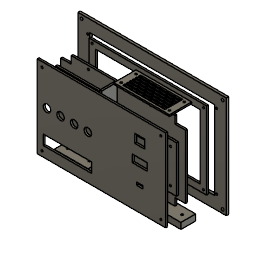
SmartMeter_Vista_Interna (Autodesk Fusion 360 design; units mm, degrees)
Autodesk Fusion 360 part; units mm, degrees
(part 1 of 2)
sketch "Esboço1" plane through (0, 0, 0) normal (0, 0, 1) x (1, 0, 0) in component "SmartMeter_DesktopFeet"
  line L0 (-102.5, -12) -> (-47.5, -12)
  line L1 (-47.5, -12) -> (-47.5, 12)
  line L2 (-47.5, 12) -> (-102.5, 12)
  line L3 (-102.5, 12) -> (-102.5, -12)
extrude "01_new_rect (1)" add sketch "Esboço1" along normal blind 10 makes body 1 in component "SmartMeter_DesktopFeet"
sketch "Esboço2" plane through (0, 0, 0) normal (0, 0, 1) x (1, 0, 0) in component "SmartMeter_DesktopFeet"
  circle A0 centre (-92.5, 0) radius 1.6
extrude "02_cut_circle (1)" cut sketch "Esboço2" along normal blind 11 bodies 1 in component "SmartMeter_DesktopFeet"
sketch "Esboço3" plane through (0, 0, 0) normal (0, 0, 1) x (1, 0, 0) in component "SmartMeter_DesktopFeet"
  circle A0 centre (-57.5, 0) radius 1.6
extrude "03_cut_circle (1)" cut sketch "Esboço3" along normal blind 11 bodies 1 in component "SmartMeter_DesktopFeet"
sketch "Esboço4" plane through (0, 0, 0) normal (0, 0, 1) x (1, 0, 0) in component "SmartMeter_DesktopFeet"
  line L0 (47.5, -12) -> (102.5, -12)
  line L1 (102.5, -12) -> (102.5, 12)
  line L2 (102.5, 12) -> (47.5, 12)
  line L3 (47.5, 12) -> (47.5, -12)
extrude "04_new_rect (1)" add sketch "Esboço4" along normal blind 10 separate body makes body 2 in component "SmartMeter_DesktopFeet"
sketch "Esboço5" plane through (0, 0, 0) normal (0, 0, 1) x (1, 0, 0) in component "SmartMeter_DesktopFeet"
  circle A0 centre (57.5, 0) radius 1.6
extrude "05_cut_circle (1)" cut sketch "Esboço5" along normal blind 11 bodies 1 2 in component "SmartMeter_DesktopFeet"
sketch "Esboço6" plane through (0, 0, 0) normal (0, 0, 1) x (1, 0, 0) in component "SmartMeter_DesktopFeet"
  circle A0 centre (92.5, 0) radius 1.6
extrude "06_cut_circle (1)" cut sketch "Esboço6" along normal blind 11 bodies 1 2 in component "SmartMeter_DesktopFeet"
sketch "Esboço1 (2)" plane through (0, 0, 0) normal (0, 0, 1) x (1, 0, 0) in component "SmartMeter_DisplayBracket"
  line L0 (-95, -62.5) -> (95, -62.5)
  line L1 (95, -62.5) -> (95, 62.5)
  line L2 (95, 62.5) -> (-95, 62.5)
  line L3 (-95, 62.5) -> (-95, -62.5)
extrude "01_new_rect (1)'" add sketch "Esboço1 (2)" along normal blind 3 separate body makes body 3 in component "SmartMeter_DisplayBracket"
sketch "Esboço2 (2)" plane through (0, 0, 0) normal (0, 0, 1) x (1, 0, 0) in component "SmartMeter_DisplayBracket"
  line L0 (-84.5, -52) -> (84.5, -52)
  line L1 (84.5, -52) -> (84.5, 52)
  line L2 (84.5, 52) -> (-84.5, 52)
  line L3 (-84.5, 52) -> (-84.5, -52)
extrude "02_cut_rect (1)" cut sketch "Esboço2 (2)" along normal blind 4 bodies 3 in component "SmartMeter_DisplayBracket"
sketch "Esboço3 (2)" plane through (0, 0, 0) normal (0, 0, 1) x (1, 0, 0) in component "SmartMeter_DisplayBracket"
  line L0 (-12, -62.5) -> (12, -62.5)
  line L1 (12, -62.5) -> (12, -52.5)
  line L2 (12, -52.5) -> (-12, -52.5)
  line L3 (-12, -52.5) -> (-12, -62.5)
extrude "03_cut_rect (1)" cut sketch "Esboço3 (2)" along normal blind 4 bodies 3 in component "SmartMeter_DisplayBracket"
sketch "Esboço4 (2)" plane through (0, 0, 0) normal (0, 0, 1) x (1, 0, 0) in component "SmartMeter_DisplayBracket"
  circle A0 centre (-90, -57.5) radius 1.6
extrude "04_cut_circle (1)" cut sketch "Esboço4 (2)" along normal blind 4 bodies 3 in component "SmartMeter_DisplayBracket"
sketch "Esboço5 (2)" plane through (0, 0, 0) normal (0, 0, 1) x (1, 0, 0) in component "SmartMeter_DisplayBracket"
  circle A0 centre (-90, 57.5) radius 1.6
extrude "05_cut_circle (1)'" cut sketch "Esboço5 (2)" along normal blind 4 bodies 3 in component "SmartMeter_DisplayBracket"
sketch "Esboço6 (2)" plane through (0, 0, 0) normal (0, 0, 1) x (1, 0, 0) in component "SmartMeter_DisplayBracket"
  circle A0 centre (90, -57.5) radius 1.6
extrude "06_cut_circle (1)'" cut sketch "Esboço6 (2)" along normal blind 4 bodies 3 in component "SmartMeter_DisplayBracket"
sketch "Esboço7" plane through (0, 0, 0) normal (0, 0, 1) x (1, 0, 0) in component "SmartMeter_DisplayBracket"
  circle A0 centre (90, 57.5) radius 1.6
extrude "07_cut_circle (1)" cut sketch "Esboço7" along normal blind 4 bodies 3 in component "SmartMeter_DisplayBracket"
sketch "Esboço1 (3)" plane through (0, 0, 0) normal (0, 0, 1) x (1, 0, 0) in component "SmartMeter_FrontPanel"
  line L0 (-102, 72.5) -> (102, 72.5)
  arc A0 (110, 64.5) -> (102, 72.5) centre (102, 64.5) ccw
  line L1 (110, 64.5) -> (110, -64.5)
  arc A1 (102, -72.5) -> (110, -64.5) centre (102, -64.5) ccw
  line L2 (102, -72.5) -> (-102, -72.5)
  arc A2 (-110, -64.5) -> (-102, -72.5) centre (-102, -64.5) ccw
  line L3 (-110, -64.5) -> (-110, 64.5)
  arc A3 (-102, 72.5) -> (-110, 64.5) centre (-102, 64.5) ccw
extrude "01_new_rounded (1)" add sketch "Esboço1 (3)" along normal blind 4 separate body makes body 4 in component "SmartMeter_FrontPanel"
sketch "Esboço2 (3)" plane through (0, 0, 0) normal (0, 0, 1) x (1, 0, 0) in component "SmartMeter_FrontPanel"
  line L0 (-77.5, -43.5) -> (77.5, -43.5)
  line L1 (77.5, -43.5) -> (77.5, 43.5)
  line L2 (77.5, 43.5) -> (-77.5, 43.5)
  line L3 (-77.5, 43.5) -> (-77.5, -43.5)
extrude "02_cut_rect (1)'" cut sketch "Esboço2 (3)" along normal blind 5 bodies 4 in component "SmartMeter_FrontPanel"
ref_plane "Plano de trabalho1" through (0, 0, 1.5) normal (0, 0, 1) x (1, 0, 0) in component "SmartMeter_FrontPanel"
sketch "Esboço3 (3)" plane through (0, 0, 1.5) normal (0, 0, 1) x (1, 0, 0) in component "SmartMeter_FrontPanel"
  line L0 (-83.5, -51) -> (83.5, -51)
  line L1 (83.5, -51) -> (83.5, 51)
  line L2 (83.5, 51) -> (-83.5, 51)
  line L3 (-83.5, 51) -> (-83.5, -51)
extrude "03_cut_rect (1)'" cut sketch "Esboço3 (3)" along normal blind 2.7 bodies 4 in component "SmartMeter_FrontPanel"
sketch "Esboço4 (3)" plane through (0, 0, 0) normal (0, 0, 1) x (1, 0, 0) in component "SmartMeter_FrontPanel"
  circle A0 centre (-90, -57.5) radius 1.6
extrude "04_cut_circle (1)'" cut sketch "Esboço4 (3)" along normal blind 5 bodies 4 in component "SmartMeter_FrontPanel"
sketch "Esboço5 (3)" plane through (0, 0, 0) normal (0, 0, 1) x (1, 0, 0) in component "SmartMeter_FrontPanel"
  circle A0 centre (-90, 57.5) radius 1.6
extrude "05_cut_circle (1)''" cut sketch "Esboço5 (3)" along normal blind 5 bodies 4 in component "SmartMeter_FrontPanel"
sketch "Esboço6 (3)" plane through (0, 0, 0) normal (0, 0, 1) x (1, 0, 0) in component "SmartMeter_FrontPanel"
  circle A0 centre (90, -57.5) radius 1.6
extrude "06_cut_circle (1)''" cut sketch "Esboço6 (3)" along normal blind 5 bodies 4 in component "SmartMeter_FrontPanel"
sketch "Esboço7 (2)" plane through (0, 0, 0) normal (0, 0, 1) x (1, 0, 0) in component "SmartMeter_FrontPanel"
  circle A0 centre (90, 57.5) radius 1.6
extrude "07_cut_circle (1)'" cut sketch "Esboço7 (2)" along normal blind 5 bodies 4 in component "SmartMeter_FrontPanel"
sketch "Esboço8" plane through (0, 0, 0) normal (0, 0, 1) x (1, 0, 0) in component "SmartMeter_FrontPanel"
  circle A0 centre (-104, -60) radius 1.6
extrude "08_cut_circle (1)" cut sketch "Esboço8" along normal blind 4 bodies 4 in component "SmartMeter_FrontPanel"
sketch "Esboço9" plane through (0, 0, 0) normal (0, 0, 1) x (1, 0, 0) in component "SmartMeter_FrontPanel"
  circle A0 centre (-104, 60) radius 1.6
extrude "09_cut_circle (1)" cut sketch "Esboço9" along normal blind 4 bodies 4 in component "SmartMeter_FrontPanel"
sketch "Esboço10" plane through (0, 0, 0) normal (0, 0, 1) x (1, 0, 0) in component "SmartMeter_FrontPanel"
  circle A0 centre (104, -60) radius 1.6
extrude "10_cut_circle (1)" cut sketch "Esboço10" along normal blind 4 bodies 4 in component "SmartMeter_FrontPanel"
sketch "Esboço11" plane through (0, 0, 0) normal (0, 0, 1) x (1, 0, 0) in component "SmartMeter_FrontPanel"
  circle A0 centre (104, 60) radius 1.6
extrude "11_cut_circle (1)" cut sketch "Esboço11" along normal blind 4 bodies 4 in component "SmartMeter_FrontPanel"
sketch "Esboço1 (4)" plane through (0, 0, 0) normal (0, 0, 1) x (1, 0, 0) in component "SmartMeter_InternalTray"
  line L0 (-101, -63.5) -> (101, -63.5)
  line L1 (101, -63.5) -> (101, 63.5)
  line L2 (101, 63.5) -> (-101, 63.5)
  line L3 (-101, 63.5) -> (-101, -63.5)
extrude "01_new_rect (1)''" add sketch "Esboço1 (4)" along normal blind 3 separate body makes body 5 in component "SmartMeter_InternalTray"
sketch "Esboço2 (4)" plane through (0, 0, 0) normal (0, 0, 1) x (1, 0, 0) in component "SmartMeter_InternalTray"
  line L0 (-12.5, -63.5) -> (-9.5, -63.5)
  line L1 (-9.5, -63.5) -> (-9.5, 63.5)
  line L2 (-9.5, 63.5) -> (-12.5, 63.5)
  line L3 (-12.5, 63.5) -> (-12.5, -63.5)
extrude "Extrusão2" add sketch "Esboço2 (4)" along normal blind 28 separate body makes body 6 in component "SmartMeter_InternalTray"
combine "02_join_rect (1)" operation add target body 5 tool bodies 6 in component "SmartMeter_InternalTray"
sketch "Esboço3 (4)" plane through (0, 0, 0) normal (0, 0, 1) x (1, 0, 0) in component "SmartMeter_InternalTray"
  circle A0 centre (-86, -30) radius 5
extrude "Extrusão3" add sketch "Esboço3 (4)" along normal blind 11 separate body makes body 7 in component "SmartMeter_InternalTray"
combine "03_join_circle (1)" operation add target body 5 tool bodies 7 in component "SmartMeter_InternalTray"
sketch "Esboço4 (4)" plane through (0, 0, 0) normal (0, 0, 1) x (1, 0, 0) in component "SmartMeter_InternalTray"
  circle A0 centre (-86, 30) radius 5
extrude "Extrusão4" add sketch "Esboço4 (4)" along normal blind 11 separate body makes body 8 in component "SmartMeter_InternalTray"
combine "04_join_circle (1)" operation add target body 5 tool bodies 8 in component "SmartMeter_InternalTray"
sketch "Esboço5 (4)" plane through (0, 0, 0) normal (0, 0, 1) x (1, 0, 0) in component "SmartMeter_InternalTray"
  circle A0 centre (-26, -30) radius 5
extrude "Extrusão5" add sketch "Esboço5 (4)" along normal blind 11 separate body makes body 9 in component "SmartMeter_InternalTray"
combine "05_join_circle (1)" operation add target body 5 tool bodies 9 in component "SmartMeter_InternalTray"
sketch "Esboço6 (4)" plane through (0, 0, 0) normal (0, 0, 1) x (1, 0, 0) in component "SmartMeter_InternalTray"
  circle A0 centre (-26, 30) radius 5
extrude "Extrusão6" add sketch "Esboço6 (4)" along normal blind 11 separate body makes body 10 in component "SmartMeter_InternalTray"
combine "06_join_circle (1)" operation add target body 5 tool bodies 10 in component "SmartMeter_InternalTray"
sketch "Esboço7 (3)" plane through (0, 0, 0) normal (0, 0, 1) x (1, 0, 0) in component "SmartMeter_InternalTray"
  circle A0 centre (10, -25) radius 5
extrude "Extrusão7" add sketch "Esboço7 (3)" along normal blind 11 separate body makes body 11 in component "SmartMeter_InternalTray"
combine "07_join_circle (1)" operation add target body 5 tool bodies 11 in component "SmartMeter_InternalTray"
sketch "Esboço8 (2)" plane through (0, 0, 0) normal (0, 0, 1) x (1, 0, 0) in component "SmartMeter_InternalTray"
  circle A0 centre (10, 25) radius 5
extrude "Extrusão8" add sketch "Esboço8 (2)" along normal blind 11 separate body makes body 12 in component "SmartMeter_InternalTray"
combine "08_join_circle (1)" operation add target body 5 tool bodies 12 in component "SmartMeter_InternalTray"
sketch "Esboço9 (2)" plane through (0, 0, 0) normal (0, 0, 1) x (1, 0, 0) in component "SmartMeter_InternalTray"
  circle A0 centre (80, -25) radius 5
extrude "Extrusão9" add sketch "Esboço9 (2)" along normal blind 11 separate body makes body 13 in component "SmartMeter_InternalTray"
combine "09_join_circle (1)" operation add target body 5 tool bodies 13 in component "SmartMeter_InternalTray"
sketch "Esboço10 (2)" plane through (0, 0, 0) normal (0, 0, 1) x (1, 0, 0) in component "SmartMeter_InternalTray"
  circle A0 centre (80, 25) radius 5
extrude "Extrusão10" add sketch "Esboço10 (2)" along normal blind 11 separate body makes body 14 in component "SmartMeter_InternalTray"
combine "10_join_circle (1)" operation add target body 5 tool bodies 14 in component "SmartMeter_InternalTray"
sketch "Esboço11 (2)" plane through (0, 0, 0) normal (0, 0, 1) x (1, 0, 0) in component "SmartMeter_InternalTray"
  line L0 (-28.5, -12) -> (-20.5, -12)
  line L1 (-20.5, -12) -> (-20.5, 12)
  line L2 (-20.5, 12) -> (-28.5, 12)
  line L3 (-28.5, 12) -> (-28.5, -12)
extrude "11_cut_rect (1)" cut sketch "Esboço11 (2)" along normal blind 3 bodies 5 in component "SmartMeter_InternalTray"
sketch "Esboço12" plane through (0, 0, 0) normal (0, 0, 1) x (1, 0, 0) in component "SmartMeter_InternalTray"
  line L0 (-1.5, -12) -> (6.5, -12)
  line L1 (6.5, -12) -> (6.5, 12)
  line L2 (6.5, 12) -> (-1.5, 12)
  line L3 (-1.5, 12) -> (-1.5, -12)
extrude "12_cut_rect (1)" cut sketch "Esboço12" along normal blind 3 bodies 5 in component "SmartMeter_InternalTray"
ref_plane "Plano de trabalho1" through (0, 0, 3) normal (0, 0, 1) x (1, 0, 0) in component "SmartMeter_InternalTray"
sketch "Esboço13" plane through (0, 0, 3) normal (0, 0, 1) x (1, 0, 0) in component "SmartMeter_InternalTray"
  circle A0 centre (-86, -30) radius 1.6
extrude "13_cut_circle (1)" cut sketch "Esboço13" along normal blind 8 bodies 5 in component "SmartMeter_InternalTray"
ref_plane "Plano de trabalho2" through (0, 0, 3) normal (0, 0, 1) x (1, 0, 0) in component "SmartMeter_InternalTray"
sketch "Esboço14" plane through (0, 0, 3) normal (0, 0, 1) x (1, 0, 0) in component "SmartMeter_InternalTray"
  circle A0 centre (-86, 30) radius 1.6
extrude "14_cut_circle (1)" cut sketch "Esboço14" along normal blind 8 bodies 5 in component "SmartMeter_InternalTray"
ref_plane "Plano de trabalho3" through (0, 0, 3) normal (0, 0, 1) x (1, 0, 0) in component "SmartMeter_InternalTray"
sketch "Esboço15" plane through (0, 0, 3) normal (0, 0, 1) x (1, 0, 0) in component "SmartMeter_InternalTray"
  circle A0 centre (-26, -30) radius 1.6
extrude "15_cut_circle (1)" cut sketch "Esboço15" along normal blind 8 bodies 5 in component "SmartMeter_InternalTray"
ref_plane "Plano de trabalho4" through (0, 0, 3) normal (0, 0, 1) x (1, 0, 0) in component "SmartMeter_InternalTray"
sketch "Esboço16" plane through (0, 0, 3) normal (0, 0, 1) x (1, 0, 0) in component "SmartMeter_InternalTray"
  circle A0 centre (-26, 30) radius 1.6
extrude "16_cut_circle (1)" cut sketch "Esboço16" along normal blind 8 bodies 5 in component "SmartMeter_InternalTray"
ref_plane "Plano de trabalho5" through (0, 0, 3) normal (0, 0, 1) x (1, 0, 0) in component "SmartMeter_InternalTray"
sketch "Esboço17" plane through (0, 0, 3) normal (0, 0, 1) x (1, 0, 0) in component "SmartMeter_InternalTray"
  circle A0 centre (10, -25) radius 1.6
extrude "17_cut_circle (1)" cut sketch "Esboço17" along normal blind 8 bodies 5 in component "SmartMeter_InternalTray"
ref_plane "Plano de trabalho6" through (0, 0, 3) normal (0, 0, 1) x (1, 0, 0) in component "SmartMeter_InternalTray"
sketch "Esboço18" plane through (0, 0, 3) normal (0, 0, 1) x (1, 0, 0) in component "SmartMeter_InternalTray"
  circle A0 centre (10, 25) radius 1.6
extrude "18_cut_circle (1)" cut sketch "Esboço18" along normal blind 8 bodies 5 in component "SmartMeter_InternalTray"
ref_plane "Plano de trabalho7" through (0, 0, 3) normal (0, 0, 1) x (1, 0, 0) in component "SmartMeter_InternalTray"
sketch "Esboço19" plane through (0, 0, 3) normal (0, 0, 1) x (1, 0, 0) in component "SmartMeter_InternalTray"
  circle A0 centre (80, -25) radius 1.6
extrude "19_cut_circle (1)" cut sketch "Esboço19" along normal blind 8 bodies 5 in component "SmartMeter_InternalTray"
ref_plane "Plano de trabalho8" through (0, 0, 3) normal (0, 0, 1) x (1, 0, 0) in component "SmartMeter_InternalTray"
sketch "Esboço20" plane through (0, 0, 3) normal (0, 0, 1) x (1, 0, 0) in component "SmartMeter_InternalTray"
  circle A0 centre (80, 25) radius 1.6
extrude "20_cut_circle (1)" cut sketch "Esboço20" along normal blind 8 bodies 5 in component "SmartMeter_InternalTray"
sketch "Esboço21" plane through (0, 0, 0) normal (0, 0, 1) x (1, 0, 0) in component "SmartMeter_InternalTray"
  line L0 (-101, -63.5) -> (-84, -63.5)
  line L1 (-84, -63.5) -> (-84, -51.5)
  line L2 (-84, -51.5) -> (-101, -51.5)
  line L3 (-101, -51.5) -> (-101, -63.5)
extrude "21_cut_rect (1)" cut sketch "Esboço21" along normal blind 3 bodies 5 in component "SmartMeter_InternalTray"
sketch "Esboço22" plane through (0, 0, 0) normal (0, 0, 1) x (1, 0, 0) in component "SmartMeter_InternalTray"
  line L0 (-101, 51.5) -> (-84, 51.5)
  line L1 (-84, 51.5) -> (-84, 63.5)
  line L2 (-84, 63.5) -> (-101, 63.5)
  line L3 (-101, 63.5) -> (-101, 51.5)
extrude "22_cut_rect (1)" cut sketch "Esboço22" along normal blind 3 bodies 5 in component "SmartMeter_InternalTray"
sketch "Esboço23" plane through (0, 0, 0) normal (0, 0, 1) x (1, 0, 0) in component "SmartMeter_InternalTray"
  line L0 (84, -63.5) -> (101, -63.5)
  line L1 (101, -63.5) -> (101, -51.5)
  line L2 (101, -51.5) -> (84, -51.5)
  line L3 (84, -51.5) -> (84, -63.5)
extrude "23_cut_rect (1)" cut sketch "Esboço23" along normal blind 3 bodies 5 in component "SmartMeter_InternalTray"
sketch "Esboço24" plane through (0, 0, 0) normal (0, 0, 1) x (1, 0, 0) in component "SmartMeter_InternalTray"
  line L0 (84, 51.5) -> (101, 51.5)
  line L1 (101, 51.5) -> (101, 63.5)
  line L2 (101, 63.5) -> (84, 63.5)
  line L3 (84, 63.5) -> (84, 51.5)
extrude "24_cut_rect (1)" cut sketch "Esboço24" along normal blind 3 bodies 5 in component "SmartMeter_InternalTray"
sketch "Esboço25" plane through (0, 0, 0) normal (0, 0, 1) x (1, 0, 0) in component "SmartMeter_InternalTray"
  circle A0 centre (-56, -58) radius 1.6
extrude "25_cut_circle (1)" cut sketch "Esboço25" along normal blind 3 bodies 5 in component "SmartMeter_InternalTray"
sketch "Esboço26" plane through (0, 0, 0) normal (0, 0, 1) x (1, 0, 0) in component "SmartMeter_InternalTray"
  circle A0 centre (-56, 58) radius 1.6
extrude "26_cut_circle (1)" cut sketch "Esboço26" along normal blind 3 bodies 5 in component "SmartMeter_InternalTray"
sketch "Esboço27" plane through (0, 0, 0) normal (0, 0, 1) x (1, 0, 0) in component "SmartMeter_InternalTray"
  circle A0 centre (45, -58) radius 1.6
extrude "27_cut_circle (1)" cut sketch "Esboço27" along normal blind 3 bodies 5 in component "SmartMeter_InternalTray"
sketch "Esboço28" plane through (0, 0, 0) normal (0, 0, 1) x (1, 0, 0) in component "SmartMeter_InternalTray"
  circle A0 centre (45, 58) radius 1.6
extrude "28_cut_circle (1)" cut sketch "Esboço28" along normal blind 3 bodies 5 in component "SmartMeter_InternalTray"
sketch "Esboço1 (5)" plane through (0, 0, 0) normal (0, 0, 1) x (1, 0, 0) in component "SmartMeter_PanelMountFrame"
  line L0 (-120, -82.5) -> (120, -82.5)
  line L1 (120, -82.5) -> (120, 82.5)
  line L2 (120, 82.5) -> (-120, 82.5)
  line L3 (-120, 82.5) -> (-120, -82.5)
extrude "01_new_rect (1)'''" add sketch "Esboço1 (5)" along normal blind 4 separate body makes body 15 in component "SmartMeter_PanelMountFrame"
sketch "Esboço2 (5)" plane through (0, 0, 0) normal (0, 0, 1) x (1, 0, 0) in component "SmartMeter_PanelMountFrame"
  line L0 (-101, -63.5) -> (101, -63.5)
  line L1 (101, -63.5) -> (101, 63.5)
  line L2 (101, 63.5) -> (-101, 63.5)
  line L3 (-101, 63.5) -> (-101, -63.5)
extrude "02_cut_rect (1)''" cut sketch "Esboço2 (5)" along normal blind 5 bodies 15 in component "SmartMeter_PanelMountFrame"
sketch "Esboço3 (5)" plane through (0, 0, 0) normal (0, 0, 1) x (1, 0, 0) in component "SmartMeter_PanelMountFrame"
  circle A0 centre (-114, -76.5) radius 2.25
extrude "03_cut_circle (1)'" cut sketch "Esboço3 (5)" along normal blind 5 bodies 15 in component "SmartMeter_PanelMountFrame"
sketch "Esboço4 (5)" plane through (0, 0, 0) normal (0, 0, 1) x (1, 0, 0) in component "SmartMeter_PanelMountFrame"
  circle A0 centre (-114, 76.5) radius 2.25
extrude "04_cut_circle (1)''" cut sketch "Esboço4 (5)" along normal blind 5 bodies 15 in component "SmartMeter_PanelMountFrame"
sketch "Esboço5 (5)" plane through (0, 0, 0) normal (0, 0, 1) x (1, 0, 0) in component "SmartMeter_PanelMountFrame"
  circle A0 centre (114, -76.5) radius 2.25
extrude "05_cut_circle (1)'''" cut sketch "Esboço5 (5)" along normal blind 5 bodies 15 in component "SmartMeter_PanelMountFrame"
sketch "Esboço6 (5)" plane through (0, 0, 0) normal (0, 0, 1) x (1, 0, 0) in component "SmartMeter_PanelMountFrame"
  circle A0 centre (114, 76.5) radius 2.25
extrude "06_cut_circle (1)'''" cut sketch "Esboço6 (5)" along normal blind 5 bodies 15 in component "SmartMeter_PanelMountFrame"
sketch "Esboço7 (4)" plane through (0, 0, 0) normal (0, 0, 1) x (1, 0, 0) in component "SmartMeter_PanelMountFrame"
  circle A0 centre (-104, -60) radius 1.6
extrude "07_cut_circle (1)''" cut sketch "Esboço7 (4)" along normal blind 4 bodies 15 in component "SmartMeter_PanelMountFrame"
sketch "Esboço8 (3)" plane through (0, 0, 0) normal (0, 0, 1) x (1, 0, 0) in component "SmartMeter_PanelMountFrame"
  circle A0 centre (-104, 60) radius 1.6
extrude "08_cut_circle (1)'" cut sketch "Esboço8 (3)" along normal blind 4 bodies 15 in component "SmartMeter_PanelMountFrame"
sketch "Esboço9 (3)" plane through (0, 0, 0) normal (0, 0, 1) x (1, 0, 0) in component "SmartMeter_PanelMountFrame"
  circle A0 centre (104, -60) radius 1.6
extrude "09_cut_circle (1)'" cut sketch "Esboço9 (3)" along normal blind 4 bodies 15 in component "SmartMeter_PanelMountFrame"
sketch "Esboço10 (3)" plane through (0, 0, 0) normal (0, 0, 1) x (1, 0, 0) in component "SmartMeter_PanelMountFrame"
  circle A0 centre (104, 60) radius 1.6
extrude "10_cut_circle (1)'" cut sketch "Esboço10 (3)" along normal blind 4 bodies 15 in component "SmartMeter_PanelMountFrame"
sketch "Esboço1 (6)" plane through (0, 0, 0) normal (0, 0, 1) x (1, 0, 0) in component "SmartMeter_RearHousing"
  line L0 (-110, -72.5) -> (110, -72.5)
  line L1 (110, -72.5) -> (110, 72.5)
  line L2 (110, 72.5) -> (-110, 72.5)
  line L3 (-110, 72.5) -> (-110, -72.5)
extrude "01_new_rect (1)''''" add sketch "Esboço1 (6)" along normal blind 75 separate body makes body 16 in component "SmartMeter_RearHousing"
sketch "Esboço2 (6)" plane through (0, 0, 0) normal (0, 0, 1) x (1, 0, 0) in component "SmartMeter_RearHousing"
  line L0 (-107, -69.5) -> (107, -69.5)
  line L1 (107, -69.5) -> (107, 69.5)
  line L2 (107, 69.5) -> (-107, 69.5)
  line L3 (-107, 69.5) -> (-107, -69.5)
extrude "02_cut_rect (1)'''" cut sketch "Esboço2 (6)" along normal blind 72 bodies 16 in component "SmartMeter_RearHousing"
ref_plane "Plano de trabalho1" through (0, 0, 3) normal (0, 0, 1) x (1, 0, 0) in component "SmartMeter_RearHousing"
sketch "Esboço3 (6)" plane through (0, 0, 3) normal (0, 0, 1) x (1, 0, 0) in component "SmartMeter_RearHousing"
  circle A0 centre (-90, -57.5) radius 5
extrude "Extrusão3'" add sketch "Esboço3 (6)" along normal blind 72 separate body makes body 17 in component "SmartMeter_RearHousing"
combine "03_join_circle (1)'" operation add target body 16 tool bodies 17 in component "SmartMeter_RearHousing"
ref_plane "Plano de trabalho2" through (0, 0, 3) normal (0, 0, 1) x (1, 0, 0) in component "SmartMeter_RearHousing"
sketch "Esboço4 (6)" plane through (0, 0, 3) normal (0, 0, 1) x (1, 0, 0) in component "SmartMeter_RearHousing"
  circle A0 centre (-90, 57.5) radius 5
extrude "Extrusão4'" add sketch "Esboço4 (6)" along normal blind 72 separate body makes body 18 in component "SmartMeter_RearHousing"
combine "04_join_circle (1)'" operation add target body 16 tool bodies 18 in component "SmartMeter_RearHousing"
ref_plane "Plano de trabalho3" through (0, 0, 3) normal (0, 0, 1) x (1, 0, 0) in component "SmartMeter_RearHousing"
sketch "Esboço5 (6)" plane through (0, 0, 3) normal (0, 0, 1) x (1, 0, 0) in component "SmartMeter_RearHousing"
  circle A0 centre (90, -57.5) radius 5
extrude "Extrusão5'" add sketch "Esboço5 (6)" along normal blind 72 separate body makes body 19 in component "SmartMeter_RearHousing"
combine "05_join_circle (1)'" operation add target body 16 tool bodies 19 in component "SmartMeter_RearHousing"
ref_plane "Plano de trabalho4" through (0, 0, 3) normal (0, 0, 1) x (1, 0, 0) in component "SmartMeter_RearHousing"
sketch "Esboço6 (6)" plane through (0, 0, 3) normal (0, 0, 1) x (1, 0, 0) in component "SmartMeter_RearHousing"
  circle A0 centre (90, 57.5) radius 5
extrude "Extrusão6'" add sketch "Esboço6 (6)" along normal blind 72 separate body makes body 20 in component "SmartMeter_RearHousing"
combine "06_join_circle (1)'" operation add target body 16 tool bodies 20 in component "SmartMeter_RearHousing"
ref_plane "Plano de trabalho5" through (0, 0, 3) normal (0, 0, 1) x (1, 0, 0) in component "SmartMeter_RearHousing"
sketch "Esboço7 (5)" plane through (0, 0, 3) normal (0, 0, 1) x (1, 0, 0) in component "SmartMeter_RearHousing"
  circle A0 centre (-90, -57.5) radius 2.3
extrude "07_cut_circle (1)'''" cut sketch "Esboço7 (5)" along normal blind 9 bodies 16 in component "SmartMeter_RearHousing"
ref_plane "Plano de trabalho6" through (0, 0, 3) normal (0, 0, 1) x (1, 0, 0) in component "SmartMeter_RearHousing"
sketch "Esboço8 (4)" plane through (0, 0, 3) normal (0, 0, 1) x (1, 0, 0) in component "SmartMeter_RearHousing"
  circle A0 centre (-90, 57.5) radius 2.3
extrude "08_cut_circle (1)''" cut sketch "Esboço8 (4)" along normal blind 9 bodies 16 in component "SmartMeter_RearHousing"
ref_plane "Plano de trabalho7" through (0, 0, 3) normal (0, 0, 1) x (1, 0, 0) in component "SmartMeter_RearHousing"
sketch "Esboço9 (4)" plane through (0, 0, 3) normal (0, 0, 1) x (1, 0, 0) in component "SmartMeter_RearHousing"
  circle A0 centre (90, -57.5) radius 2.3
extrude "09_cut_circle (1)''" cut sketch "Esboço9 (4)" along normal blind 9 bodies 16 in component "SmartMeter_RearHousing"
ref_plane "Plano de trabalho8" through (0, 0, 3) normal (0, 0, 1) x (1, 0, 0) in component "SmartMeter_RearHousing"
sketch "Esboço10 (4)" plane through (0, 0, 3) normal (0, 0, 1) x (1, 0, 0) in component "SmartMeter_RearHousing"
  circle A0 centre (90, 57.5) radius 2.3
extrude "10_cut_circle (1)''" cut sketch "Esboço10 (4)" along normal blind 9 bodies 16 in component "SmartMeter_RearHousing"
ref_plane "Plano de trabalho9" through (0, 0, 72) normal (0, 0, 1) x (1, 0, 0) in component "SmartMeter_RearHousing"
sketch "Esboço11 (3)" plane through (0, 0, 72) normal (0, 0, 1) x (1, 0, 0) in component "SmartMeter_RearHousing"
  line L0 (-94, -50) -> (-16, -50)
  line L1 (-16, -50) -> (-16, -34)
  line L2 (-16, -34) -> (-94, -34)
  line L3 (-94, -34) -> (-94, -50)
extrude "11_cut_rect (1)'" cut sketch "Esboço11 (3)" along normal blind 4 bodies 16 in component "SmartMeter_RearHousing"
ref_plane "Plano de trabalho10" through (0, 0, 72) normal (0, 0, 1) x (1, 0, 0) in component "SmartMeter_RearHousing"
sketch "Esboço12 (2)" plane through (0, 0, 72) normal (0, 0, 1) x (1, 0, 0) in component "SmartMeter_RearHousing"
  circle A0 centre (-88, 5) radius 6
extrude "12_cut_circle (1)" cut sketch "Esboço12 (2)" along normal blind 4 bodies 16 in component "SmartMeter_RearHousing"
ref_plane "Plano de trabalho11" through (0, 0, 72) normal (0, 0, 1) x (1, 0, 0) in component "SmartMeter_RearHousing"
sketch "Esboço13 (2)" plane through (0, 0, 72) normal (0, 0, 1) x (1, 0, 0) in component "SmartMeter_RearHousing"
  circle A0 centre (-66, 5) radius 6
extrude "13_cut_circle (1)'" cut sketch "Esboço13 (2)" along normal blind 4 bodies 16 in component "SmartMeter_RearHousing"
ref_plane "Plano de trabalho12" through (0, 0, 72) normal (0, 0, 1) x (1, 0, 0) in component "SmartMeter_RearHousing"
sketch "Esboço14 (2)" plane through (0, 0, 72) normal (0, 0, 1) x (1, 0, 0) in component "SmartMeter_RearHousing"
  circle A0 centre (-44, 5) radius 6
extrude "14_cut_circle (1)'" cut sketch "Esboço14 (2)" along normal blind 4 bodies 16 in component "SmartMeter_RearHousing"
ref_plane "Plano de trabalho13" through (0, 0, 72) normal (0, 0, 1) x (1, 0, 0) in component "SmartMeter_RearHousing"
sketch "Esboço15 (2)" plane through (0, 0, 72) normal (0, 0, 1) x (1, 0, 0) in component "SmartMeter_RearHousing"
  circle A0 centre (-22, 5) radius 6
extrude "15_cut_circle (1)'" cut sketch "Esboço15 (2)" along normal blind 4 bodies 16 in component "SmartMeter_RearHousing"
ref_plane "Plano de trabalho14" through (0, 0, 72) normal (0, 0, 1) x (1, 0, 0) in component "SmartMeter_RearHousing"
sketch "Esboço16 (2)" plane through (0, 0, 72) normal (0, 0, 1) x (1, 0, 0) in component "SmartMeter_RearHousing"
  line L0 (54, 27) -> (70, 27)
  line L1 (70, 27) -> (70, 41)
  line L2 (70, 41) -> (54, 41)
  line L3 (54, 41) -> (54, 27)
extrude "16_cut_rect (1)" cut sketch "Esboço16 (2)" along normal blind 4 bodies 16 in component "SmartMeter_RearHousing"
ref_plane "Plano de trabalho15" through (0, 0, 72) normal (0, 0, 1) x (1, 0, 0) in component "SmartMeter_RearHousing"
sketch "Esboço17 (2)" plane through (0, 0, 72) normal (0, 0, 1) x (1, 0, 0) in component "SmartMeter_RearHousing"
  line L0 (50, -2) -> (74, -2)
  line L1 (74, -2) -> (74, 10)
  line L2 (74, 10) -> (50, 10)
  line L3 (50, 10) -> (50, -2)
extrude "17_cut_rect (1)" cut sketch "Esboço17 (2)" along normal blind 4 bodies 16 in component "SmartMeter_RearHousing"
ref_plane "Plano de trabalho16" through (0, 0, 72) normal (0, 0, 1) x (1, 0, 0) in component "SmartMeter_RearHousing"
sketch "Esboço18 (2)" plane through (0, 0, 72) normal (0, 0, 1) x (1, 0, 0) in component "SmartMeter_RearHousing"
  line L0 (57, -30.25) -> (67, -30.25)
  line L1 (67, -30.25) -> (67, -25.75)
  line L2 (67, -25.75) -> (57, -25.75)
  line L3 (57, -25.75) -> (57, -30.25)
extrude "18_cut_rect (1)" cut sketch "Esboço18 (2)" along normal blind 4 bodies 16 in component "SmartMeter_RearHousing"
ref_plane "Plano de trabalho17" through (0, 0, 72) normal (0, 0, 1) x (1, 0, 0) in component "SmartMeter_RearHousing"
sketch "Esboço19 (2)" plane through (0, 0, 72) normal (0, 0, 1) x (1, 0, 0) in component "SmartMeter_RearHousing"
  circle A0 centre (-96, -58.5) radius 1.6
extrude "19_cut_circle (1)'" cut sketch "Esboço19 (2)" along normal blind 4 bodies 16 in component "SmartMeter_RearHousing"
ref_plane "Plano de trabalho18" through (0, 0, 72) normal (0, 0, 1) x (1, 0, 0) in component "SmartMeter_RearHousing"
sketch "Esboço20 (2)" plane through (0, 0, 72) normal (0, 0, 1) x (1, 0, 0) in component "SmartMeter_RearHousing"
  circle A0 centre (-96, 58.5) radius 1.6
extrude "20_cut_circle (1)'" cut sketch "Esboço20 (2)" along normal blind 4 bodies 16 in component "SmartMeter_RearHousing"
ref_plane "Plano de trabalho19" through (0, 0, 72) normal (0, 0, 1) x (1, 0, 0) in component "SmartMeter_RearHousing"
sketch "Esboço21 (2)" plane through (0, 0, 72) normal (0, 0, 1) x (1, 0, 0) in component "SmartMeter_RearHousing"
  circle A0 centre (96, -58.5) radius 1.6
extrude "21_cut_circle (1)" cut sketch "Esboço21 (2)" along normal blind 4 bodies 16 in component "SmartMeter_RearHousing"
ref_plane "Plano de trabalho20" through (0, 0, 72) normal (0, 0, 1) x (1, 0, 0) in component "SmartMeter_RearHousing"
sketch "Esboço22 (2)" plane through (0, 0, 72) normal (0, 0, 1) x (1, 0, 0) in component "SmartMeter_RearHousing"
  circle A0 centre (96, 58.5) radius 1.6
extrude "22_cut_circle (1)" cut sketch "Esboço22 (2)" along normal blind 4 bodies 16 in component "SmartMeter_RearHousing"
ref_plane "Plano de trabalho21" through (0, 0, 43) normal (0, 0, 1) x (1, 0, 0) in component "SmartMeter_RearHousing"
sketch "Esboço23 (2)" plane through (0, 0, 43) normal (0, 0, 1) x (1, 0, 0) in component "SmartMeter_RearHousing"
  circle A0 centre (-56, -58) radius 5
extrude "Extrusão23" add sketch "Esboço23 (2)" along normal blind 32 separate body makes body 21 in component "SmartMeter_RearHousing"
combine "23_join_circle (1)" operation add target body 16 tool bodies 21 in component "SmartMeter_RearHousing"
ref_plane "Plano de trabalho22" through (0, 0, 43) normal (0, 0, 1) x (1, 0, 0) in component "SmartMeter_RearHousing"
sketch "Esboço24 (2)" plane through (0, 0, 43) normal (0, 0, 1) x (1, 0, 0) in component "SmartMeter_RearHousing"
  circle A0 centre (-56, -58) radius 2.3
extrude "24_cut_circle (1)" cut sketch "Esboço24 (2)" along normal blind 9 bodies 16 in component "SmartMeter_RearHousing"
ref_plane "Plano de trabalho23" through (0, 0, 43) normal (0, 0, 1) x (1, 0, 0) in component "SmartMeter_RearHousing"
sketch "Esboço25 (2)" plane through (0, 0, 43) normal (0, 0, 1) x (1, 0, 0) in component "SmartMeter_RearHousing"
  circle A0 centre (-56, 58) radius 5
extrude "Extrusão25" add sketch "Esboço25 (2)" along normal blind 32 separate body makes body 22 in component "SmartMeter_RearHousing"
combine "25_join_circle (1)" operation add target body 16 tool bodies 22 in component "SmartMeter_RearHousing"
ref_plane "Plano de trabalho24" through (0, 0, 43) normal (0, 0, 1) x (1, 0, 0) in component "SmartMeter_RearHousing"
sketch "Esboço26 (2)" plane through (0, 0, 43) normal (0, 0, 1) x (1, 0, 0) in component "SmartMeter_RearHousing"
  circle A0 centre (-56, 58) radius 2.3
extrude "26_cut_circle (1)'" cut sketch "Esboço26 (2)" along normal blind 9 bodies 16 in component "SmartMeter_RearHousing"
ref_plane "Plano de trabalho25" through (0, 0, 43) normal (0, 0, 1) x (1, 0, 0) in component "SmartMeter_RearHousing"
sketch "Esboço27 (2)" plane through (0, 0, 43) normal (0, 0, 1) x (1, 0, 0) in component "SmartMeter_RearHousing"
  circle A0 centre (45, -58) radius 5
extrude "Extrusão27" add sketch "Esboço27 (2)" along normal blind 32 separate body makes body 23 in component "SmartMeter_RearHousing"
combine "27_join_circle (1)" operation add target body 16 tool bodies 23 in component "SmartMeter_RearHousing"
ref_plane "Plano de trabalho26" through (0, 0, 43) normal (0, 0, 1) x (1, 0, 0) in component "SmartMeter_RearHousing"
sketch "Esboço28 (2)" plane through (0, 0, 43) normal (0, 0, 1) x (1, 0, 0) in component "SmartMeter_RearHousing"
  circle A0 centre (45, -58) radius 2.3
extrude "28_cut_circle (1)'" cut sketch "Esboço28 (2)" along normal blind 9 bodies 16 in component "SmartMeter_RearHousing"
ref_plane "Plano de trabalho27" through (0, 0, 43) normal (0, 0, 1) x (1, 0, 0) in component "SmartMeter_RearHousing"
sketch "Esboço29" plane through (0, 0, 43) normal (0, 0, 1) x (1, 0, 0) in component "SmartMeter_RearHousing"
  circle A0 centre (45, 58) radius 5
extrude "Extrusão29" add sketch "Esboço29" along normal blind 32 separate body makes body 24 in component "SmartMeter_RearHousing"
combine "29_join_circle (1)" operation add target body 16 tool bodies 24 in component "SmartMeter_RearHousing"
ref_plane "Plano de trabalho28" through (0, 0, 43) normal (0, 0, 1) x (1, 0, 0) in component "SmartMeter_RearHousing"
sketch "Esboço30" plane through (0, 0, 43) normal (0, 0, 1) x (1, 0, 0) in component "SmartMeter_RearHousing"
  circle A0 centre (45, 58) radius 2.3
extrude "30_cut_circle (1)" cut sketch "Esboço30" along normal blind 9 bodies 16 in component "SmartMeter_RearHousing"
sketch "Esboço31" plane through (0, 0, 0) normal (0, 0, 1) x (1, 0, 0) in component "SmartMeter_RearHousing"
  circle A0 centre (-104, -60) radius 4
extrude "Extrusão31" add sketch "Esboço31" along normal blind 75 separate body makes body 25 in component "SmartMeter_RearHousing"
combine "31_join_circle (1)" operation add target body 16 tool bodies 25 in component "SmartMeter_RearHousing"
sketch "Esboço32" plane through (0, 0, 0) normal (0, 0, 1) x (1, 0, 0) in component "SmartMeter_RearHousing"
  circle A0 centre (-104, -60) radius 2.3
extrude "32_cut_circle (1)" cut sketch "Esboço32" along normal blind 9 bodies 16 in component "SmartMeter_RearHousing"
sketch "Esboço33" plane through (0, 0, 0) normal (0, 0, 1) x (1, 0, 0) in component "SmartMeter_RearHousing"
  circle A0 centre (-104, 60) radius 4
extrude "Extrusão33" add sketch "Esboço33" along normal blind 75 separate body makes body 26 in component "SmartMeter_RearHousing"
combine "33_join_circle (1)" operation add target body 16 tool bodies 26 in component "SmartMeter_RearHousing"
sketch "Esboço34" plane through (0, 0, 0) normal (0, 0, 1) x (1, 0, 0) in component "SmartMeter_RearHousing"
  circle A0 centre (-104, 60) radius 2.3
extrude "34_cut_circle (1)" cut sketch "Esboço34" along normal blind 9 bodies 16 in component "SmartMeter_RearHousing"
sketch "Esboço35" plane through (0, 0, 0) normal (0, 0, 1) x (1, 0, 0) in component "SmartMeter_RearHousing"
  circle A0 centre (104, -60) radius 4
extrude "Extrusão35" add sketch "Esboço35" along normal blind 75 separate body makes body 27 in component "SmartMeter_RearHousing"
combine "35_join_circle (1)" operation add target body 16 tool bodies 27 in component "SmartMeter_RearHousing"
sketch "Esboço36" plane through (0, 0, 0) normal (0, 0, 1) x (1, 0, 0) in component "SmartMeter_RearHousing"
  circle A0 centre (104, -60) radius 2.3
extrude "36_cut_circle (1)" cut sketch "Esboço36" along normal blind 9 bodies 16 in component "SmartMeter_RearHousing"
sketch "Esboço37" plane through (0, 0, 0) normal (0, 0, 1) x (1, 0, 0) in component "SmartMeter_RearHousing"
  circle A0 centre (104, 60) radius 4
extrude "Extrusão37" add sketch "Esboço37" along normal blind 75 separate body makes body 28 in component "SmartMeter_RearHousing"
combine "37_join_circle (1)" operation add target body 16 tool bodies 28 in component "SmartMeter_RearHousing"
sketch "Esboço38" plane through (0, 0, 0) normal (0, 0, 1) x (1, 0, 0) in component "SmartMeter_RearHousing"
  circle A0 centre (104, 60) radius 2.3
extrude "38_cut_circle (1)" cut sketch "Esboço38" along normal blind 9 bodies 16 in component "SmartMeter_RearHousing"
ref_plane "Plano de trabalho29" through (0, 69.5, 0) normal (0, 1, 0) x (0, 0, 1) in component "SmartMeter_RearHousing"
sketch "Esboço39" plane through (0, 69.5, 0) normal (0, 1, 0) x (1, 0, 0) in component "SmartMeter_RearHousing"
  circle A0 through (-90.9, -40, -139) (-93.3, -38.6144, -139) (-93.3, -41.3856, -139)
extrude "39_cut_circle (1)" cut sketch "Esboço39" along normal blind 4 contours A0 in plane through (0, -69.5, 0) normal (0, 1, 0) bodies 16 in component "SmartMeter_RearHousing"
ref_plane "Plano de trabalho30" through (0, 69.5, 0) normal (0, 1, 0) x (0, 0, 1) in component "SmartMeter_RearHousing"
sketch "Esboço40" plane through (0, 69.5, 0) normal (0, 1, 0) x (1, 0, 0) in component "SmartMeter_RearHousing"
  circle A0 through (-55.9, -40, -139) (-58.3, -38.6144, -139) (-58.3, -41.3856, -139)
extrude "40_cut_circle (1)" cut sketch "Esboço40" along normal blind 4 contours A0 in plane through (0, -69.5, 0) normal (0, 1, 0) bodies 16 in component "SmartMeter_RearHousing"
ref_plane "Plano de trabalho31" through (0, 69.5, 0) normal (0, 1, 0) x (0, 0, 1) in component "SmartMeter_RearHousing"
sketch "Esboço41" plane through (0, 69.5, 0) normal (0, 1, 0) x (1, 0, 0) in component "SmartMeter_RearHousing"
  circle A0 through (59.1, -40, -139) (56.7, -38.6144, -139) (56.7, -41.3856, -139)
extrude "41_cut_circle (1)" cut sketch "Esboço41" along normal blind 4 contours A0 in plane through (0, -69.5, 0) normal (0, 1, 0) bodies 16 in component "SmartMeter_RearHousing"
ref_plane "Plano de trabalho32" through (0, 69.5, 0) normal (0, 1, 0) x (0, 0, 1) in component "SmartMeter_RearHousing"
sketch "Esboço42" plane through (0, 69.5, 0) normal (0, 1, 0) x (1, 0, 0) in component "SmartMeter_RearHousing"
  circle A0 through (94.1, -40, -139) (91.7, -38.6144, -139) (91.7, -41.3856, -139)
extrude "42_cut_circle (1)" cut sketch "Esboço42" along normal blind 4 contours A0 in plane through (0, -69.5, 0) normal (0, 1, 0) bodies 16 in component "SmartMeter_RearHousing"
ref_plane "Plano de trabalho33" through (0, -72.5, 0) normal (0, 1, 0) x (0, 0, 1) in component "SmartMeter_RearHousing"
sketch "Esboço43" plane through (0, -72.5, 0) normal (0, 1, 0) x (1, 0, 0) in component "SmartMeter_RearHousing"
  line L0 (9, -25, 145) -> (81, -25, 145)
  line L1 (81, -25, 145) -> (81, -55, 145)
  line L2 (81, -55, 145) -> (9, -55, 145)
  line L3 (9, -55, 145) -> (9, -25, 145)
extrude "43_cut_rect (1)" cut sketch "Esboço43" along normal blind 3.5 contours L0 L1 L2 L3 in plane through (0, 72.5, 0) normal (0, 1, 0) bodies 16 in component "SmartMeter_RearHousing"
ref_plane "Plano de trabalho34" through (0, -72.5, 0) normal (0, 1, 0) x (0, 0, 1) in component "SmartMeter_RearHousing"
sketch "Esboço44" plane through (0, -72.5, 0) normal (0, 1, 0) x (1, 0, 0) in component "SmartMeter_RearHousing"
  circle A0 through (7.6, -28, 145) (5.2, -26.6144, 145) (5.2, -29.3856, 145)
extrude "44_cut_circle (1)" cut sketch "Esboço44" along normal blind 3.5 contours A0 in plane through (0, 72.5, 0) normal (0, 1, 0) bodies 16 in component "SmartMeter_RearHousing"
ref_plane "Plano de trabalho35" through (0, -72.5, 0) normal (0, 1, 0) x (0, 0, 1) in component "SmartMeter_RearHousing"
sketch "Esboço45" plane through (0, -72.5, 0) normal (0, 1, 0) x (1, 0, 0) in component "SmartMeter_RearHousing"
  circle A0 through (7.6, -52, 145) (5.2, -50.6144, 145) (5.2, -53.3856, 145)
extrude "45_cut_circle (1)" cut sketch "Esboço45" along normal blind 3.5 contours A0 in plane through (0, 72.5, 0) normal (0, 1, 0) bodies 16 in component "SmartMeter_RearHousing"
ref_plane "Plano de trabalho36" through (0, -72.5, 0) normal (0, 1, 0) x (0, 0, 1) in component "SmartMeter_RearHousing"
sketch "Esboço46" plane through (0, -72.5, 0) normal (0, 1, 0) x (1, 0, 0) in component "SmartMeter_RearHousing"
  circle A0 through (85.6, -28, 145) (83.2, -26.6144, 145) (83.2, -29.3856, 145)
extrude "46_cut_circle (1)" cut sketch "Esboço46" along normal blind 3.5 contours A0 in plane through (0, 72.5, 0) normal (0, 1, 0) bodies 16 in component "SmartMeter_RearHousing"
ref_plane "Plano de trabalho37" through (0, -72.5, 0) normal (0, 1, 0) x (0, 0, 1) in component "SmartMeter_RearHousing"
sketch "Esboço47" plane through (0, -72.5, 0) normal (0, 1, 0) x (1, 0, 0) in component "SmartMeter_RearHousing"
  circle A0 through (85.6, -52, 145) (83.2, -50.6144, 145) (83.2, -53.3856, 145)
extrude "47_cut_circle (1)" cut sketch "Esboço47" along normal blind 3.5 contours A0 in plane through (0, 72.5, 0) normal (0, 1, 0) bodies 16 in component "SmartMeter_RearHousing"
sketch "Esboço1 (7)" plane through (0, 0, 0) normal (0, 0, 1) x (1, 0, 0) in component "SmartMeter_RearPanel"
  line L0 (-104, -66.5) -> (104, -66.5)
  line L1 (104, -66.5) -> (104, 66.5)
  line L2 (104, 66.5) -> (-104, 66.5)
  line L3 (-104, 66.5) -> (-104, -66.5)
extrude "01_new_rect (1)'''''" add sketch "Esboço1 (7)" along normal blind 3 separate body makes body 29 in component "SmartMeter_RearPanel"
sketch "Esboço2 (7)" plane through (0, 0, 0) normal (0, 0, 1) x (1, 0, 0) in component "SmartMeter_RearPanel"
  line L0 (-94, -50) -> (-16, -50)
  line L1 (-16, -50) -> (-16, -34)
  line L2 (-16, -34) -> (-94, -34)
  line L3 (-94, -34) -> (-94, -50)
extrude "02_cut_rect (1)''''" cut sketch "Esboço2 (7)" along normal blind 4 bodies 29 in component "SmartMeter_RearPanel"
sketch "Esboço3 (7)" plane through (0, 0, 0) normal (0, 0, 1) x (1, 0, 0) in component "SmartMeter_RearPanel"
  circle A0 centre (-88, 5) radius 6
extrude "03_cut_circle (1)''" cut sketch "Esboço3 (7)" along normal blind 4 bodies 29 in component "SmartMeter_RearPanel"
sketch "Esboço4 (7)" plane through (0, 0, 0) normal (0, 0, 1) x (1, 0, 0) in component "SmartMeter_RearPanel"
  circle A0 centre (-66, 5) radius 6
extrude "04_cut_circle (1)'''" cut sketch "Esboço4 (7)" along normal blind 4 bodies 29 in component "SmartMeter_RearPanel"
sketch "Esboço5 (7)" plane through (0, 0, 0) normal (0, 0, 1) x (1, 0, 0) in component "SmartMeter_RearPanel"
  circle A0 centre (-44, 5) radius 6
extrude "05_cut_circle (1)''''" cut sketch "Esboço5 (7)" along normal blind 4 bodies 29 in component "SmartMeter_RearPanel"
sketch "Esboço6 (7)" plane through (0, 0, 0) normal (0, 0, 1) x (1, 0, 0) in component "SmartMeter_RearPanel"
  circle A0 centre (-22, 5) radius 6
extrude "06_cut_circle (1)''''" cut sketch "Esboço6 (7)" along normal blind 4 bodies 29 in component "SmartMeter_RearPanel"
sketch "Esboço7 (6)" plane through (0, 0, 0) normal (0, 0, 1) x (1, 0, 0) in component "SmartMeter_RearPanel"
  line L0 (54, 27) -> (70, 27)
  line L1 (70, 27) -> (70, 41)
  line L2 (70, 41) -> (54, 41)
  line L3 (54, 41) -> (54, 27)
extrude "07_cut_rect (1)" cut sketch "Esboço7 (6)" along normal blind 4 bodies 29 in component "SmartMeter_RearPanel"
sketch "Esboço8 (5)" plane through (0, 0, 0) normal (0, 0, 1) x (1, 0, 0) in component "SmartMeter_RearPanel"
  line L0 (50, -2) -> (74, -2)
  line L1 (74, -2) -> (74, 10)
  line L2 (74, 10) -> (50, 10)
  line L3 (50, 10) -> (50, -2)
extrude "08_cut_rect (1)" cut sketch "Esboço8 (5)" along normal blind 4 bodies 29 in component "SmartMeter_RearPanel"
sketch "Esboço9 (5)" plane through (0, 0, 0) normal (0, 0, 1) x (1, 0, 0) in component "SmartMeter_RearPanel"
  line L0 (57, -30.25) -> (67, -30.25)
  line L1 (67, -30.25) -> (67, -25.75)
  line L2 (67, -25.75) -> (57, -25.75)
  line L3 (57, -25.75) -> (57, -30.25)
extrude "09_cut_rect (1)" cut sketch "Esboço9 (5)" along normal blind 4 bodies 29 in component "SmartMeter_RearPanel"
sketch "Esboço10 (5)" plane through (0, 0, 0) normal (0, 0, 1) x (1, 0, 0) in component "SmartMeter_RearPanel"
  circle A0 centre (-96, -58.5) radius 1.6
extrude "10_cut_circle (1)'''" cut sketch "Esboço10 (5)" along normal blind 4 bodies 29 in component "SmartMeter_RearPanel"
sketch "Esboço11 (4)" plane through (0, 0, 0) normal (0, 0, 1) x (1, 0, 0) in component "SmartMeter_RearPanel"
  circle A0 centre (-96, 58.5) radius 1.6
extrude "11_cut_circle (1)'" cut sketch "Esboço11 (4)" along normal blind 4 bodies 29 in component "SmartMeter_RearPanel"
sketch "Esboço12 (3)" plane through (0, 0, 0) normal (0, 0, 1) x (1, 0, 0) in component "SmartMeter_RearPanel"
  circle A0 centre (96, -58.5) radius 1.6
extrude "12_cut_circle (1)'" cut sketch "Esboço12 (3)" along normal blind 4 bodies 29 in component "SmartMeter_RearPanel"
sketch "Esboço13 (3)" plane through (0, 0, 0) normal (0, 0, 1) x (1, 0, 0) in component "SmartMeter_RearPanel"
  circle A0 centre (96, 58.5) radius 1.6
extrude "13_cut_circle (1)''" cut sketch "Esboço13 (3)" along normal blind 4 bodies 29 in component "SmartMeter_RearPanel"
sketch "Esboço1 (8)" plane through (0, 0, 0) normal (0, 0, 1) x (1, 0, 0) in component "SmartMeter_VentilationGrille"
  line L0 (-45, -18) -> (45, -18)
  line L1 (45, -18) -> (45, 18)
  line L2 (45, 18) -> (-45, 18)
  line L3 (-45, 18) -> (-45, -18)
extrude "01_new_rect (1)''''''" add sketch "Esboço1 (8)" along normal blind 2.5 separate body makes body 30 in component "SmartMeter_VentilationGrille"
sketch "Esboço2 (8)" plane through (0, 0, 0) normal (0, 0, 1) x (1, 0, 0) in component "SmartMeter_VentilationGrille"
  line L0 (-34, -14.25) -> (34, -14.25)
  line L1 (34, -14.25) -> (34, -10.75)
  line L2 (34, -10.75) -> (-34, -10.75)
  line L3 (-34, -10.75) -> (-34, -14.25)
extrude "02_cut_rect (1)'''''" cut sketch "Esboço2 (8)" along normal blind 3.5 bodies 30 in component "SmartMeter_VentilationGrille"
sketch "Esboço3 (8)" plane through (0, 0, 0) normal (0, 0, 1) x (1, 0, 0) in component "SmartMeter_VentilationGrille"
  line L0 (-34, -9.25) -> (34, -9.25)
  line L1 (34, -9.25) -> (34, -5.75)
  line L2 (34, -5.75) -> (-34, -5.75)
  line L3 (-34, -5.75) -> (-34, -9.25)
extrude "03_cut_rect (1)''" cut sketch "Esboço3 (8)" along normal blind 3.5 bodies 30 in component "SmartMeter_VentilationGrille"
sketch "Esboço4 (8)" plane through (0, 0, 0) normal (0, 0, 1) x (1, 0, 0) in component "SmartMeter_VentilationGrille"
  line L0 (-34, -4.25) -> (34, -4.25)
  line L1 (34, -4.25) -> (34, -0.75)
  line L2 (34, -0.75) -> (-34, -0.75)
  line L3 (-34, -0.75) -> (-34, -4.25)
extrude "04_cut_rect (1)" cut sketch "Esboço4 (8)" along normal blind 3.5 bodies 30 in component "SmartMeter_VentilationGrille"
sketch "Esboço5 (8)" plane through (0, 0, 0) normal (0, 0, 1) x (1, 0, 0) in component "SmartMeter_VentilationGrille"
  line L0 (-34, 0.75) -> (34, 0.75)
  line L1 (34, 0.75) -> (34, 4.25)
  line L2 (34, 4.25) -> (-34, 4.25)
  line L3 (-34, 4.25) -> (-34, 0.75)
extrude "05_cut_rect (1)" cut sketch "Esboço5 (8)" along normal blind 3.5 bodies 30 in component "SmartMeter_VentilationGrille"
sketch "Esboço6 (8)" plane through (0, 0, 0) normal (0, 0, 1) x (1, 0, 0) in component "SmartMeter_VentilationGrille"
  line L0 (-34, 5.75) -> (34, 5.75)
  line L1 (34, 5.75) -> (34, 9.25)
  line L2 (34, 9.25) -> (-34, 9.25)
  line L3 (-34, 9.25) -> (-34, 5.75)
extrude "06_cut_rect (1)" cut sketch "Esboço6 (8)" along normal blind 3.5 bodies 30 in component "SmartMeter_VentilationGrille"
sketch "Esboço7 (7)" plane through (0, 0, 0) normal (0, 0, 1) x (1, 0, 0) in component "SmartMeter_VentilationGrille"
  line L0 (-34, 10.75) -> (34, 10.75)
  line L1 (34, 10.75) -> (34, 14.25)
  line L2 (34, 14.25) -> (-34, 14.25)
  line L3 (-34, 14.25) -> (-34, 10.75)
extrude "07_cut_rect (1)'" cut sketch "Esboço7 (7)" along normal blind 3.5 bodies 30 in component "SmartMeter_VentilationGrille"
sketch "Esboço8 (6)" plane through (0, 0, 0) normal (0, 0, 1) x (1, 0, 0) in component "SmartMeter_VentilationGrille"
  circle A0 centre (-39, -12) radius 1.6
extrude "08_cut_circle (1)'''" cut sketch "Esboço8 (6)" along normal blind 3.5 bodies 30 in component "SmartMeter_VentilationGrille"
sketch "Esboço9 (6)" plane through (0, 0, 0) normal (0, 0, 1) x (1, 0, 0) in component "SmartMeter_VentilationGrille"
  circle A0 centre (-39, 12) radius 1.6
extrude "09_cut_circle (1)'''" cut sketch "Esboço9 (6)" along normal blind 3.5 bodies 30 in component "SmartMeter_VentilationGrille"
sketch "Esboço10 (6)" plane through (0, 0, 0) normal (0, 0, 1) x (1, 0, 0) in component "SmartMeter_VentilationGrille"
  circle A0 centre (39, -12) radius 1.6
extrude "10_cut_circle (1)''''" cut sketch "Esboço10 (6)" along normal blind 3.5 bodies 30 in component "SmartMeter_VentilationGrille"